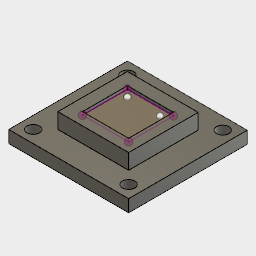
IUMSensorMount v2 (Autodesk Fusion 360 design; units mm, degrees)
Autodesk Fusion 360 part; units mm, degrees
sketch "Sketch1" plane through (0, 0, 0) normal (0, 1, 0) x (1, 0, 0)
  line L0 (-55.88, 25.4) -> (-36.83, 25.4)
  line L1 (-36.83, 25.4) -> (-36.83, 6.858)
  line L2 (-36.83, 6.858) -> (-55.88, 6.858)
  line L3 (-55.88, 6.858) -> (-55.88, 25.4)
  dimension "d1" = 19.05
  dimension "d2" = 18.542
  constraint horizontal L0
  constraint vertical L1
  constraint horizontal L2
  constraint vertical L3
  measures "d1" distance of origin
  measures "d2" distance of origin
  measures "d30" distance of L1
  measures "d31" distance of L1
extrude "Extrude1" add sketch "Sketch1" along normal blind 10.16
sketch "Sketch2" plane through (0, 0, 0) normal (0, -1, 0) x (1, 0, 0)
  line L0 (-36.83, -6.858) -> (-55.88, -6.858)
  line L1 (-55.88, -6.858) -> (-55.88, -25.4)
  line L2 (-55.88, -25.4) -> (-36.83, -25.4)
  line L3 (-36.83, -25.4) -> (-36.83, -6.858)
  line L4 (-60.96, -1.778) -> (-31.75, -1.778)
  line L5 (-31.75, -1.778) -> (-31.75, -30.48)
  line L6 (-31.75, -30.48) -> (-60.96, -30.48)
  line L7 (-60.96, -30.48) -> (-60.96, -1.778)
  dimension "d5" = 5.08
  dimension "d6" = 5.08
  dimension "d7" = 5.08
  dimension "d8" = 5.08
  constraint horizontal L4
  constraint vertical L5
  constraint horizontal L6
  constraint vertical L7
  measures "d5" distance of L1 L7
  measures "d6" distance of L3 L5
  measures "d7" distance of L0 L4
  measures "d8" distance of L2 L6
extrude "Extrude2" add sketch "Sketch2" against normal blind 11.43
sketch "Sketch3" plane through (0, 0, 0) normal (0, -1, 0) x (1, 0, 0)
  line L0 (-60.96, -30.48) -> (-31.75, -30.48)
  line L1 (-31.75, -30.48) -> (-31.75, -1.778)
  line L2 (-31.75, -1.778) -> (-60.96, -1.778)
  line L3 (-60.96, -1.778) -> (-60.96, -30.48)
  line L4 (-71.12, 8.382) -> (-21.59, 8.382)
  line L5 (-21.59, 8.382) -> (-21.59, -40.64)
  line L6 (-21.59, -40.64) -> (-71.12, -40.64)
  line L7 (-71.12, -40.64) -> (-71.12, 8.382)
  dimension "d11" = 10.16
  dimension "d12" = 10.16
  dimension "d13" = 10.16
  dimension "d14" = 10.16
  constraint horizontal L4
  constraint vertical L5
  constraint horizontal L6
  constraint vertical L7
  measures "d13" distance of L0 L6
extrude "Extrude3" add sketch "Sketch3" against normal blind 5.08
sketch "Sketch4" plane through (0, 5.08, 0) normal (0, 1, 0) x (-1, 0, 0)
  line L0 (60.96, -1.778) -> (60.96, -30.48)
  line L1 (60.96, -30.48) -> (31.75, -30.48)
  line L2 (31.75, -30.48) -> (31.75, -1.778)
  line L3 (31.75, -1.778) -> (60.96, -1.778)
  line L4 (21.59, -40.64) -> (71.12, -40.64)
  line L5 (71.12, -40.64) -> (71.12, 8.382)
  line L6 (71.12, 8.382) -> (21.59, 8.382)
  line L7 (21.59, 8.382) -> (21.59, -40.64)
  dimension "d17" = 5.08
  dimension "d18" = 5.08
  dimension "d19" = 5.08
  dimension "d20" = 5.08
  dimension "d21" = 5.08
  dimension "d22" = 5.08
  dimension "d23" = 5.08
  dimension "d24" = 5.08
hole "Hole1" at (-66.04, 5.08, -35.56) at (-26.67, 5.08, -35.56) at (-26.67, 5.08, 3.302) at (-66.04, 5.08, 3.302) direction (0, -1, 0) diameter 5.08 depth 17.78 tip angle 118
sketch "Sketch5" plane through (0, 10.16, 0) normal (0, 1, 0) x (-1, 0, 0)
  line L0 (55.88, -6.858) -> (36.83, -6.858)
  line L1 (36.83, -6.858) -> (36.83, -25.4)
  line L2 (36.83, -25.4) -> (55.88, -25.4)
  line L3 (55.88, -25.4) -> (55.88, -6.858)
  line L4 (36.83, -6.858) -> (55.88, -6.858)
  line L5 (36.83, -25.4) -> (36.83, -6.858)
  line L6 (55.88, -25.4) -> (36.83, -25.4)
  line L7 (55.88, -6.858) -> (55.88, -25.4)
  dimension "d30" = 2.794
  dimension "d31" = 2.794
  dimension "d35" = 2.794
  dimension "d36" = 2.794
  measures "d30" distance of origin L5
  measures "d31" distance of origin L6
  measures "d35" distance of origin L6
hole "Hole2" [suppressed]
